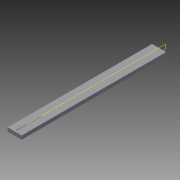
# Autodesk Inventor part: 16 Drawer Slide
Saved by Autodesk Inventor 2014 SP2 (Build 180246200, 246)
## iProperties
Created: 2014-09-12
Part Number: 16 Drawer Slide
Material: Generic
Document SubType Name: Modeling
Designer: Allison
Density: 1 g/cm^3
Appearance: Default
Author: Allison
Autodesk Inventor part; units mm, degrees
ref_plane "YZ Plane" through (0, 0, 0) normal (1, 0, 0) x (0, 1, 0)
ref_plane "XZ Plane" through (0, 0, 0) normal (0, 1, 0) x (-1, 0, 0)
ref_plane "XY Plane" through (0, 0, 0) normal (0, 0, 1) x (1, 0, 0)
sketch "Sketch1" plane through (0, 0, 0) normal (0, 0, 1) x (1, 0, 0)
  line L0 (0, 0) -> (44.45, 0)
  line L1 (44.45, 0) -> (44.45, 11.43)
  line L2 (44.45, 11.43) -> (0, 11.43)
  line L3 (0, 11.43) -> (0, 0)
  dimension "d0" = 44.45
  dimension "d1" = 11.43
  constraints: 8 end point, 2 parallel, 1 horizontal, 1 perpendicular
  measures "d0" distance of L2.end L1.end
  measures "d1" distance of L1.end L0.end
extrude "Extrusion1" add sketch "Sketch1" along normal blind 457.2
ref_plane "Work Plane1" through (22.225, 0, 0) normal (1, 0, 0) x (0, 0, -1)
sketch "Sketch2" plane through (0, 11.43, 0) normal (0, 1, 0) x (1, 0, 0)
  circle A0 centre (22.225, -448.9182) radius 1.8542
  dimension "d4" = 3.7084
  constraints: 1 centre point
  measures "d4" diameter of A0
extrude "Extrusion2" cut sketch "Sketch2" against normal blind 25.4
pattern_linear "Rectangular Pattern1" count 15 spacing 5.334 along (0, 0, -1) of "Extrusion2"
body "Solid1"
